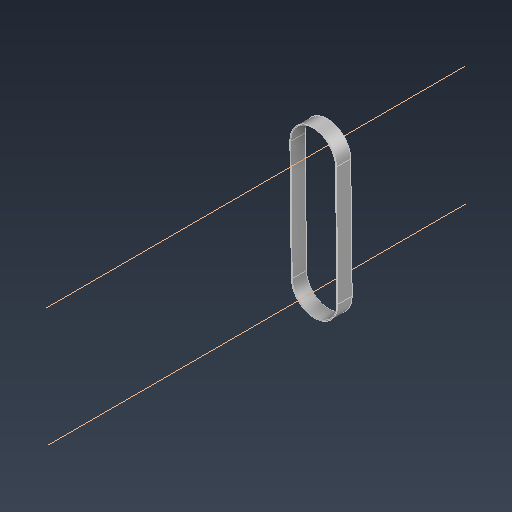
# Autodesk Inventor part: Зубчатый ремень
Saved by Autodesk Inventor 2025 (Build 290162000, 162)
## iProperties
Created: 2025-09-22
Part Number: Зубчатый ремень
Material: Rubber
Document SubType Name: Modeling
Designer: GameHD
Density: 1 g/cm^3
Appearance: Rubber - Black - Version 1.1
CustomPartVersion: 1
Author: GameHD
Autodesk Inventor part; units mm, degrees
sketch "Эскизная траектория" plane through (0, 0, 0) normal (0, 0, 1) x (1, 0, 0)
  arc A0 (-16.0494, -0.2501) -> (15.7793, 0.1314) centre (-0.1351, -0.0594) ccw
  arc A1 (14.7905, 82.6254) -> (-17.0382, 82.2439) centre (-1.1239, 82.4347) ccw
  line L0 (14.7905, 82.6254) -> (15.7793, 0.1314)
  line L1 (-16.0494, -0.2501) -> (-17.0382, 82.2439)
  constraints: 4 end point, 4 point on circle, 2 centre point
ref_plane "Плоскость сечения" through (15.7793, 0.1314, 0) normal (-0.012, 0.9999, 0) x (0, 0, 1)
ref_plane "РабПлоскость2" through (-0.1351, -0.0594, 0) normal (-1, 0, 0) x (0, 0, 1)
ref_plane "РабПлоскость3" through (-1.1239, 82.4347, 0) normal (0, -1, 0) x (0, 0, 1)
sketch "Сечение" plane through (15.7793, 0.1314, 0) normal (-0.012, 0.9999, 0) x (0, 0, 1)
  line L0 (-5, 0.3) -> (5, 0.3)
  line L1 (5, 0.3) -> (5, -0.3)
  line L2 (5, -0.3) -> (-5, -0.3)
  line L3 (-5, -0.3) -> (-5, 0.3)
  line L4 (-5, 0) -> (5, 0) construction
  point P0 (0, 0)
  point P1 (0, 0)
  dimension "d0" = 10
  dimension "d4" = 0.3
  dimension "d5" = 0.3
  constraints: 10 end point, 3 midpoint, 2 parallel, 1 coincident, 1 horizontal, 1 perpendicular, 1 other
  measures "d0" distance between parallel lines of L1 L3
  measures "d4" distance between parallel lines of L2 L4
  measures "d5" distance between parallel lines of L4 L0
sweep "Ремень" add profiles "Сечение" path "Эскизная траектория"
equation "\"d0\" = da_B"
equation "\"d4\" = da_a"
equation "\"d5\" = da_a2"
equation "\"da_B\" = 10"
equation "\"da_pb\" = 2.5"
equation "\"da_L\" = 265"
equation "\"da_a\" = 0.3"
equation "\"da_S\" = 1.5"
equation "\"da_Beta\" = 20deg"
equation "\"da_Ht\" = 0.7"
equation "\"da_H\" = 2"
equation "\"da_a2\" = 0.3"
body "Solid1"
